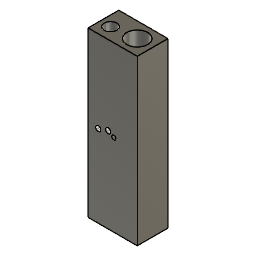
heat_block_als_tool (Autodesk Fusion 360 design; units mm, degrees)
Autodesk Fusion 360 part; units mm, degrees
note: some values were not read from the file. Set by a fixed rule: the direction of a hole.
sketch "Sketch1" plane through (0, 0, 0) normal (0, 1, 0) x (1, 0, 0)
  line L0 (0, 0) -> (-24, 0)
  line L1 (-24, 0) -> (-24, -80)
  line L2 (-24, -80) -> (0, -80)
  line L3 (0, -80) -> (0, 0)
  line L4 (-2.4, -80) -> (-2.4, 0) construction
  line L5 (-12.6, 0) -> (-12.6, -80) construction
  line L6 (-22.05, 0) -> (-22.05, -80) construction
  line L7 (-15.95, 0) -> (-15.95, -80) construction
  line L8 (-12.6, -40) -> (-2.4, -40) construction
  line L9 (-7.5, -40) -> (-7.5, 0) construction
  line L10 (-22.05, -40) -> (-15.95, -40) construction
  line L11 (-22.05, -40) -> (-24, -40) construction
  line L12 (-2.4, -40) -> (0, -40) construction
  line L13 (-12.6, -5) -> (-2.4, -5) construction
  line L14 (-14.2, -41.5) -> (-11.4, -41.5) construction
  line L15 (-11.4, -41.5) -> (-11.4, -40) construction
  line L16 (-11.4, -40) -> (-14.2, -40) construction
  line L17 (-14.2, -40) -> (-14.2, -41.5) construction
  point P0 (-19, -40)
  point P1 (-14.2, -41.5)
  point P2 (-11.4, -40)
  dimension "d1" = 24
  dimension "d2" = 80
  dimension "d3" = 10.2
  dimension "d5" = 6.1
  dimension "d7" = 5
  dimension "d8" = 7.5
  dimension "d9" = 75
  dimension "d12" = 1.5
  dimension "d13" = 2.8
  dimension "d14" = 1.2
  constraint horizontal L0
  constraint vertical L1
  constraint horizontal L2
  constraint vertical L3
  constraint coincident L0.start L3.end
  constraint coincident L2 L4.start
  constraint coincident L0 L4.end
  constraint perpendicular L0 L4
  constraint coincident L0 L5.start
  constraint coincident L2 L5.end
  constraint perpendicular L2 L5
  constraint coincident L0 L6.start
  constraint coincident L2 L6.end
  constraint perpendicular L2 L6
  constraint coincident L0 L7.start
  constraint coincident L2 L7.end
  constraint perpendicular L0 L7
  constraint midpoint L5 L8.start
  constraint midpoint L4 L8.end
  constraint midpoint L8 L9.start
  constraint coincident L0 L9.end
  constraint perpendicular L0 L9
  constraint midpoint L6 L10.start
  constraint midpoint L7 L10.end
  constraint midpoint L10 P0
  constraint midpoint L1 L11.end
  constraint midpoint L3 L12.end
  constraint coincident L5 L13.start
  constraint coincident L4 L13.end
  constraint perpendicular L4 L13
  constraint horizontal L14
  constraint vertical L15
  constraint horizontal L16
  constraint vertical L17
  constraint coincident P1 L14.start
  constraint coincident P2 L15.end
  constraint coincident L8 P2
  measures "d1" distance of L0.start L0.end
  measures "d2" distance of L0.start L2.end
  measures "d3" distance of L8.start L8.end
  measures "d5" distance of L10.start L10.end
  measures "d7" distance of P0 L11.end
  measures "d8" distance of L9.start L12.end
  measures "d9" distance of L4.start L13.end
  measures "d12" distance of L14.end P2
  measures "d13" distance of P2 L16.end
  measures "d14" distance of L8.start P2
extrude "Extrude1" add sketch "Sketch1" along normal blind 15
sketch "Sketch2" plane through (0, 0, 80) normal (0, 0, 1) x (-1, 0, 0)
  line L0 (24, 0) -> (0, 0)
  line L1 (0, 0) -> (0, -15)
  line L2 (0, -15) -> (24, -15)
  line L3 (24, -15) -> (24, 0)
  line L4 (15.95, 0) -> (15.95, -15) construction
  line L5 (22.05, 0) -> (22.05, -15) construction
  line L6 (12.6, 0) -> (12.6, -15) construction
  line L7 (2.4, 0) -> (2.4, -15) construction
  line L8 (12.6, -7.5) -> (2.4, -7.5) construction
  line L9 (15.95, -6) -> (22.05, -6) construction
  circle A0 centre (7.5, -7.5) radius 5.1
  circle A1 centre (19, -6) radius 3.05
  point P0 (22.05, 0)
  point P1 (15.95, 0)
  point P2 (12.6, 0)
  point P3 (2.4, 0)
  point P4 (19, 0)
  dimension "d15" = 6
  constraint coincident P1 L4.start
  constraint coincident L2 L4.end
  constraint perpendicular L2 L4
  constraint coincident P0 L5.start
  constraint coincident L2 L5.end
  constraint perpendicular L2 L5
  constraint coincident P2 L6.start
  constraint coincident L2 L6.end
  constraint perpendicular L2 L6
  constraint coincident P3 L7.start
  constraint coincident L2 L7.end
  constraint perpendicular L2 L7
  constraint midpoint L6 L8.start
  constraint midpoint L7 L8.end
  constraint coincident L4 L9.start
  constraint coincident L5 L9.end
  constraint perpendicular L5 L9
  constraint midpoint L8 A0.centre
  constraint coincident L8.start A0
  constraint midpoint L9 A1.centre
  constraint coincident L9.end A1
  measures "d15" distance of A1.centre P4
extrude "Extrude2" cut sketch "Sketch2" against normal through all contours A1
hole "Hole1" at (-7.5, 7.5, 80) direction (0, 0, -1) diameter 10.2 depth 75 tip angle 118
hole "Hole2" at (-14.2, 0, 41.5) direction (0, 1, 0) diameter 2.529 depth 8 tip angle 118
thread "Thread1" "ISO Metric profile 3.0 M3x0.5 M3x0.5 6H" thread offset 0 thread depth 7.2
hole "Hole3" at (-19, 0, 40) direction (0, 1, 0) diameter 2.529 depth 6 tip angle 118
thread "Thread2" "ISO Metric profile 3.0 M3x0.5 M3x0.5 6H" thread offset 0 thread depth 7.2
hole "Hole4" at (-11.4, 0, 40) direction (0, 1, 0) diameter 2 depth 3 tip angle 118
